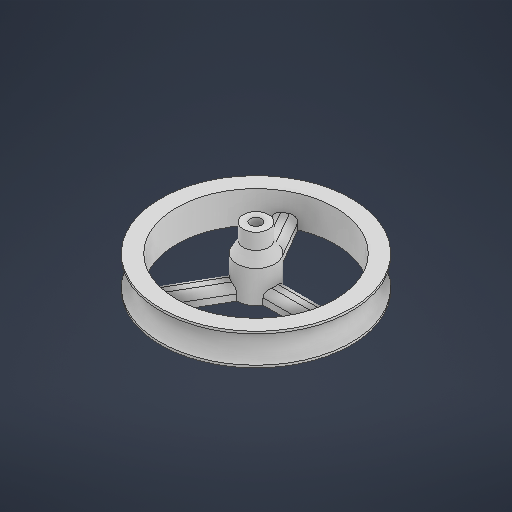
# Autodesk Inventor part: Koło
Saved by Autodesk Inventor 2026 (Build 300175000, 175)
## iProperties
Created: 2025-04-24
Part Number: Koło
Material: Generic
Document SubType Name: Modeling
Designer: isan
Density: 1 g/cm^3
Appearance: Default
Author: isan
Autodesk Inventor part; units mm, degrees
ref_plane "YZ Plane" through (0, 0, 0) normal (1, 0, 0) x (0, 1, 0)
ref_plane "XZ Plane" through (0, 0, 0) normal (0, 1, 0) x (-1, 0, 0)
ref_plane "XY Plane" through (0, 0, 0) normal (0, 0, 1) x (1, 0, 0)
sketch "Sketch1" plane through (0, 0, 0) normal (0, 0, 1) x (1, 0, 0)
  circle A0 centre (0, 0) radius 15
  circle A1 centre (0, 0) radius 12.5
  dimension "d0" = 30
  dimension "d1" = 25
  constraints: 2 centre point, 2 coincident
  measures "d0" diameter of A0
  measures "d1" diameter of A1
extrude "Extrusion1" add sketch "Sketch1" along normal blind 5
sketch "Sketch2" plane through (0, 0, 0) normal (0, 0, -1) x (-1, 0, 0)
  circle A0 centre (0, 0) radius 3
  dimension "d5" = 6
  constraints: 1 centre point, 1 coincident
  measures "d5" diameter of A0
extrude "Extrusion2" add sketch "Sketch2" against normal blind 6.8
sketch "Sketch3" plane through (0, 0, 6.8) normal (0, 0, 1) x (1, 0, 0)
  circle A0 centre (0, 0) radius 2
  dimension "d8" = 4
  constraints: 1 centre point, 1 coincident
  measures "d8" diameter of A0
extrude "Extrusion3" add sketch "Sketch3" along normal blind 2.5
chamfer "Chamfer1" distance 1 angle 60 1 edges at (3, 0, 6.8) measured on face at (2.5, 0, 6.8)
sketch "Sketch4" plane through (0, 0, 9.3) normal (0, 0, 1) x (1, 0, 0)
  circle A0 centre (0, 0) radius 0.9
  dimension "d14" = 1.8
  constraints: 1 centre point, 1 coincident
  measures "d14" diameter of A0
extrude "Extrusion4" cut sketch "Sketch4" against normal blind 4.8
sketch "Sketch5" plane through (0, 0, 0) normal (0, 0, -1) x (-1, 0, 0)
  line L0 (-2, 1.5) -> (-13, 1.5)
  line L1 (-13, 1.5) -> (-13, -1.5)
  line L2 (-13, -1.5) -> (-2, -1.5)
  line L3 (-2, -1.5) -> (-2, 1.5)
  circle A0 centre (0, 0) radius 0.9 projected
  line L4 (0, 0) -> (-17.4633, 0) construction
  circle A1 centre (0, 0) radius 3
  circle A2 centre (0, 0) radius 12.5
  point P0 (-13, 0)
  point P1 (-12.4097, 1.5)
  point P2 (-12.4097, -1.5)
  point P3 (-2.5981, -1.5)
  point P4 (-2.5981, 1.5)
  dimension "d19" = 3
  dimension "d20" = 11
  constraints: 10 end point, 2 centre point, 2 coincident, 2 horizontal, 2 parallel, 1 midpoint, 1 perpendicular, 1 point on line
  measures "d19" distance of L0.end L1.end
  measures "d20" distance of L0.start L0.end
extrude "Extrusion6" add sketch "Sketch5" against normal blind 2 contours A1 L2 A2 L0 picked at (-9.3212, 0.1045)
pattern_circular "Circular Pattern2" count 3 over 360 about axis through (0, 0, -10) along (0, 0, 1) of "Extrusion6"
sketch "Sketch6" plane through (0, 0, 4.5) normal (0, 0, 1) x (1, 0, 0)
  circle A0 centre (0, 0) radius 2 projected
  circle A1 centre (0, 0) radius 0.4
  dimension "d32" = 0.8
  constraints: 1 centre point, 1 coincident
  measures "d32" diameter of A1
extrude "Extrusion7" cut sketch "Sketch6" against normal blind 5.3 contours A1
sketch "Sketch7" plane through (0, 0, 0) normal (0, 1, 0) x (-1, 0, 0)
  point P0 (0, 0)
sketch "Sketch8" plane through (0, 0, 0) normal (0, 1, 0) x (-1, 0, 0)
  line L0 (15, 0) -> (15, 5) projected
  circle A0 centre (16.3, 2.5) radius 2.5
  line L1 (0, 0) -> (0, 2) projected
  line L2 (0, 0) -> (0, 12.0754) construction
  point P0 (15, 2.5)
  point P1 (15, 4.6354)
  point P2 (15, 0.3646)
  dimension "d35" = 5
  dimension "d36" = 1.3
  constraints: 2 end point, 1 centre point, 1 midpoint, 1 vertical
  measures "d35" diameter of A0
  measures "d36" distance of point (15, 2.5) A0.centre
revolve "Revolution1" cut sketch "Sketch8" angle 360 about axis through (0, 0, 0) along (0, 0, 1)
fillet "Fillet1" radius 1 6 edges at (-5.051, 5.7485, 2) (-2.4529, 7.2485, 2) (-5.051, -5.7485, 2) (-2.4529, -7.2485, 2) (7.5039, -1.5, 2) (7.5039, 1.5, 2)
body "Solid1"
